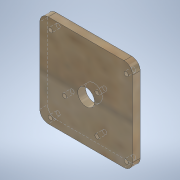
# Autodesk Inventor part: 前後直動12x12_4
Saved by Autodesk Inventor 2020.3 (Build 243373000, 373)
## iProperties
Created: 2020-07-05
Part Number: 前後直動12x12_4
Material: 木材 (カエデ材)
Document SubType Name: Modeling
Designer: totot
Density: 0.67 g/cm^3
Appearance: ナチュラル カエデ材 - 光沢 濃い着色
Mass: 15.3389 g
Surface Area: 102.906 cm^2
Volume: 22.8939 cm^3
Author: totot
Autodesk Inventor part; units mm, degrees
ref_plane "YZ Plane" through (0, 0, 0) normal (1, 0, 0) x (0, 1, 0)
ref_plane "XZ Plane" through (0, 0, 0) normal (0, 1, 0) x (-1, 0, 0)
ref_plane "XY Plane" through (0, 0, 0) normal (0, 0, 1) x (1, 0, 0)
sketch "スケッチ1" plane through (0, 0, 0) normal (0, 0, 1) x (1, 0, 0)
  line L0 (0, 0) -> (66, 0)
  line L1 (66, 0) -> (66, -66)
  line L2 (66, -66) -> (0, -66)
  line L3 (0, -66) -> (0, 0)
  dimension "d0" = 66
  dimension "d1" = 66
  constraints: 8 end point, 2 parallel, 1 horizontal, 1 perpendicular
  measures "d0" distance of L1.end L2.end
  measures "d1" distance of L0.end L1.end
extrude "押し出し1" add sketch "スケッチ1" along normal blind 5.5
sketch "スケッチ2" plane through (0, 0, 5.5) normal (0, 0, 1) x (1, 0, 0)
  line L0 (66, 0) -> (0, 0) projected
  line L1 (0, 0) -> (0, -66) projected
  point P0 (7.5, -7.5)
  point P1 (61.5, -7.5)
  point P2 (61.5, -61.5)
  point P3 (7.5, -61.5)
  dimension "d4" = 7.5
  dimension "d5" = 7.5
  dimension "d6" = 7.5
  dimension "d7" = 54
  dimension "d8" = 54
  dimension "d9" = 54
  dimension "d10" = 54
  dimension "d19" = 7.5
  measures "d4" distance from line of point (7.5, -7.5) L0
  measures "d5" distance from line of point (7.5, -7.5) L1
  measures "d6" distance from line of L0 point (61.5, -7.5)
  measures "d7" distance of point (61.5, -7.5) point (7.5, -7.5)
  measures "d8" distance of point (7.5, -61.5) point (7.5, -7.5)
  measures "d9" distance of point (61.5, -7.5) point (61.5, -61.5)
  measures "d10" distance of point (7.5, -61.5) point (61.5, -61.5)
  measures "d19" distance from line of L1 point (7.5, -61.5)
hole "穴1" at (7.5, -7.5, 5.5) at (61.5, -7.5, 5.5) at (61.5, -61.5, 5.5) at (7.5, -61.5, 5.5) direction (0, 0, -1) diameter 3 end through all
fillet "フィレット1" radius 6 4 edges at (66, 0, 2.75) (66, -66, 2.75) (0, 0, 2.75) (0, -66, 2.75)
sketch "スケッチ3" plane through (0, 0, 0) normal (0, 0, -1) x (-1, 0, 0)
  circle A0 centre (-33, -43) radius 15.5
  line L0 (-66, -60) -> (-66, -6) projected
  line L1 (0, -6) -> (0, -60) projected
  line L2 (-60, 0) -> (-6, 0) projected
  line L3 (-6, -66) -> (-60, -66) projected
  line L4 (-33, -43) -> (-17.5, -43)
  line L5 (-33, -43) -> (-40.75, -29.5766)
  line L6 (-33, -43) -> (-40.75, -56.4234)
  point P0 (0, 0)
  dimension "d20" = 31
  dimension "d21" = 33
  dimension "d22" = 66
  dimension "d23" = 66
  dimension "d24" = 23
  dimension "d25" = 120
  dimension "d26" = 120
  constraints: 6 end point, 3 coincident, 3 point on circle, 1 centre point, 1 horizontal
  measures "d20" diameter of A0
  measures "d21" distance from line of L4.start L0
  measures "d22" distance between parallel lines of L0 L1
  measures "d23" distance between parallel lines of L2 L3
  measures "d24" distance from line of L4.start L3
  measures "d25" angle of L5 L4
  measures "d26" angle of L5 L6
hole "穴2" at (40.75, -56.4234, 0) at (40.75, -29.5766, 0) at (17.5, -43, 0) direction (0, 0, 1) diameter 3 end through all
sketch "スケッチ4" plane through (0, 0, 0) normal (0, 0, -1) x (-1, 0, 0)
  line L0 (-33, -43) -> (-33, -36)
  line L1 (-6, -66) -> (-60, -66) projected
  line L2 (-60, 0) -> (-6, 0) projected
  line L3 (-66, -60) -> (-66, -6) projected
  point P0 (0, 0)
  dimension "d34" = 7
  dimension "d35" = 23
  dimension "d36" = 66
  dimension "d37" = 33
  constraints: 2 end point, 1 coincident, 1 vertical
  measures "d34" distance of L0.start L0.end
  measures "d35" distance from line of L0.start L1
  measures "d36" distance between parallel lines of L2 L1
  measures "d37" distance between parallel lines of L0 L3
hole "穴3" at (33, -36, 0) direction (0, 0, 1) diameter 12 end through all
equation "\"d4\" = d5"
equation "\"d5\" = d19"
equation "\"d6\" = d4"
equation "\"d10\" = d7"
equation "\"d21\" = 0.5 * d22"
